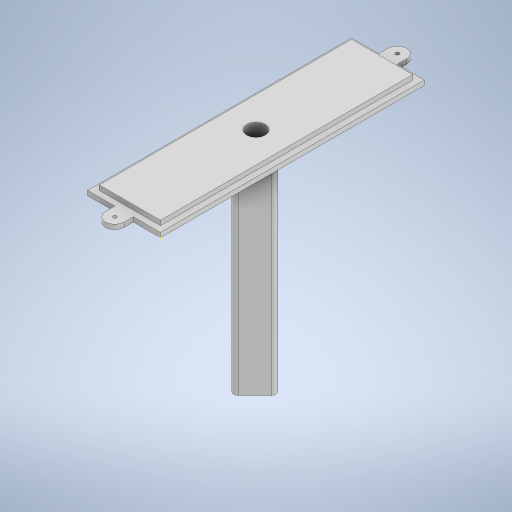
# Autodesk Inventor part: Tampa Suporte 4E
Saved by Autodesk Inventor 2023 (Build 270158000, 158)
## iProperties
Created: 2023-03-29
Part Number: Tampa Suporte 4E
Material: Genérico
Document SubType Name: Modeling
Designer: Inteli
Density: 1 g/cm^3
Appearance: Padrão
Author: Inteli
## iProperties of the stored document Tampa Suporte 4E_3DPrint.ipt
Created: 2023-03-29
Part Number: Tampa Suporte 4E_3DPrint
Material: Genérico
Document SubType Name: Modeling
Designer: Inteli
Density: 1 g/cm^3
Appearance: Padrão
Author: Inteli
Autodesk Inventor part; units mm, degrees
ref_plane "YZ Plane" through (0, 0, 0) normal (1, 0, 0) x (0, 1, 0)
ref_plane "XZ Plane" through (0, 0, 0) normal (0, 1, 0) x (-1, 0, 0)
ref_plane "XY Plane" through (0, 0, 0) normal (0, 0, 1) x (1, 0, 0)
sketch "Esboço1" plane through (0, 0, 0) normal (0, 1, 0) x (-1, 0, 0)
  line L0 (0, 0) -> (31.3, 0)
  line L1 (31.3, 0) -> (31.3, -113.5)
  line L2 (31.3, -113.5) -> (0, -113.5)
  line L3 (0, -113.5) -> (0, 0)
  line L4 (28.8, -111) -> (28.8, -2.5)
  line L5 (28.8, -2.5) -> (2.5, -2.5)
  line L6 (2.5, -2.5) -> (2.5, -111)
  line L7 (2.5, -111) -> (28.8, -111)
  dimension "d0" = 31.3
  dimension "d1" = 113.5
  dimension "d2" = 2.5
  constraints: 16 end point, 4 parallel, 2 perpendicular, 1 horizontal, 3 other
  measures "d0" distance of L1.end L2.end
  measures "d1" distance of L0.end L1.end
  measures "d2" distance between parallel lines of L1 L4
extrude "Extrusão1" add sketch "Esboço1" along normal blind 2 contours L7 L6 L5 L4
extrude "Extrusão2" add sketch "Esboço1" against normal blind 2 contours L0 L1 L2 L3 | L7 L6 L5 L4
sketch "Esboço2" plane through (0, -2, 0) normal (0, -1, 0) x (1, 0, 0)
  line L0 (0, -113.5) -> (0, 0) projected
  line L1 (-15.65, 0) -> (-11.65, 0)
  line L2 (-11.65, 0) -> (-11.65, 4)
  line L3 (-19.65, 0) -> (-15.65, 0)
  line L4 (-28.8, -2.5) -> (-2.5, -2.5) projected
  circle A0 centre (-15.65, 4) radius 0.8
  line L5 (0, 0) -> (0, -113.5) projected
  line L6 (-19.65, 0) -> (-19.65, 4)
  arc A1 (-11.65, 4) -> (-19.65, 4) centre (-15.65, 4) ccw
  line L7 (-31.3, -113.5) -> (-31.3, 0) projected
  line L8 (-15.65, -113.5) -> (-11.65, -113.5)
  line L9 (-11.65, -113.5) -> (-11.65, -117.5)
  line L10 (-19.65, -113.5) -> (-15.65, -113.5)
  circle A2 centre (-15.65, -117.5) radius 0.8
  line L11 (-19.65, -113.5) -> (-19.65, -117.5)
  arc A3 (-19.65, -117.5) -> (-11.65, -117.5) centre (-15.65, -117.5) ccw
  dimension "d16" = 1.6
  dimension "d28" = 0
  constraints: 16 end point, 4 centre point, 4 point on circle, 2 tangent, 1 parallel, 1 vertical
  measures "d16" diameter of A0
  measures "d28" distance of A1.centre A0.centre
extrude "Extrusão3" add sketch "Esboço2" against normal blind 2
sketch "Esboço3" plane through (0, -2, 0) normal (0, -1, 0) x (1, 0, 0)
  circle A0 centre (-15.65, -56.75) radius 4
  line L0 (0, -113.5) -> (0, 0) projected
  line L1 (-31.3, 0) -> (-31.3, -113.5) projected
  line L2 (0, -113.5) -> (-31.3, -113.5) projected
  dimension "d18" = 8
  dimension "d21" = 15.65
  dimension "d33" = 56.75
  constraints: 1 centre point
  measures "d18" diameter of A0
  measures "d21" distance from line of A0.centre L0
  measures "d33" distance from line of A0.centre L2
extrude "Extrusão4" cut sketch "Esboço3" against normal up to surface (4 mm away)
sketch "Esboço4" plane through (0, -2, 0) normal (0, -1, 0) x (1, 0, 0)
  circle A0 centre (-15.65, 4) radius 0.8 projected
  circle A1 centre (-15.65, 4) radius 2.6
  line L0 (0, -113.5) -> (0, 0) projected
  circle A2 centre (-15.65, -117.5) radius 2.6
  dimension "d29" = 5.2
  constraints: 2 centre point, 1 coincident
  measures "d29" diameter of A1
extrude "Extrusão5" cut sketch "Esboço4" against normal blind 1
sketch "Esboço5" plane through (0, -2, 0) normal (0, -1, 0) x (1, 0, 0)
  point P0 (0, 0)
sketch "Esboço6" plane through (0, -2, 0) normal (0, -1, 0) x (1, 0, 0)
  line L0 (-17.3312, -47.9978) -> (-24.4022, -55.0688)
  line L1 (-24.4022, -57.8973) -> (-17.3312, -64.9683)
  line L2 (-14.5027, -64.9683) -> (-7.4317, -57.8973)
  line L3 (-7.4317, -55.0688) -> (-14.5027, -47.9978)
  circle A0 centre (-15.65, -56.75) radius 4 projected
  line L4 (-15.917, -46.5835) -> (-15.917, -66.3825) construction
  line L5 (-25.8165, -56.483) -> (-6.0175, -56.483) construction
  arc A1 (-24.4022, -55.0688) -> (-24.4022, -57.8973) centre (-22.988, -56.483) ccw
  arc A2 (-17.3312, -64.9683) -> (-14.5027, -64.9683) centre (-15.917, -63.5541) ccw
  arc A3 (-7.4317, -57.8973) -> (-7.4317, -55.0688) centre (-8.8459, -56.483) ccw
  arc A4 (-14.5027, -47.9978) -> (-17.3312, -47.9978) centre (-15.917, -49.412) ccw
  point P0 (0, 0)
  dimension "d34" = 14
  dimension "d35" = 2
  dimension "d38" = 14
  constraints: 12 end point, 8 point on circle, 8 point on line, 8 tangent, 4 centre point, 3 equal radius, 2 parallel, 1 perpendicular
  measures "d34" distance of L5.end L4.end
  measures "d35" radius of A1
  measures "d38" distance between parallel lines of L0 L2
extrude "Extrusão6" add sketch "Esboço6" along normal blind 90
